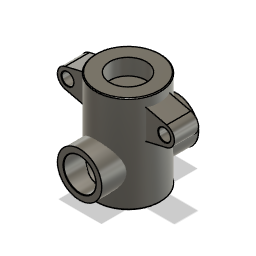
wheel hub v1 (Autodesk Fusion 360 design; units mm, degrees)
Autodesk Fusion 360 part; units mm, degrees
sketch "Sketch1" plane through (0, 0, 0) normal (0, 0, 1) x (1, 0, 0)
  line L0 (0, 0) -> (40, 0)
  line L1 (40, 0) -> (40, 120)
  line L2 (40, 120) -> (0, 120)
  line L3 (0, 120) -> (0, 0)
  dimension "d1" = 40
  dimension "d2" = 120
  constraint horizontal L0
  constraint vertical L1
  constraint horizontal L2
  constraint vertical L3
  constraint coincident L0.start L3.end
  measures "d1" distance of L1.end L2.end
  measures "d2" distance of L0.end L1.end
revolve "Revolve1" add sketch "Sketch1" angle 360 about axis through (0, 120, 0) along (0, -1, 0) makes body 1
sketch "Sketch2" plane through (0, 0, 0) normal (0, 0, 1) x (1, 0, 0)
sketch "Sketch3" plane through (0, 0, 0) normal (0, 0, 1) x (1, 0, 0)
  line L0 (0, 150) -> (0, -10) construction
  line L1 (-70, 90) -> (60, 90) construction
  line L2 (30, 110) -> (30, 70)
  line L3 (30, 70) -> (62.898, 77.8406)
  line L4 (30, 110) -> (62.898, 102.1594)
  circle A0 centre (60, 90) radius 7.5
  arc A1 (62.898, 77.8406) -> (62.898, 102.1594) centre (60, 90) ccw
  point P0 (40, 120)
  dimension "d4" = 25
  dimension "d5" = 20
  dimension "d6" = 40
  dimension "d7" = 10
  dimension "d8" = 15
  constraint vertical L0
  constraint perpendicular L0 L1
  constraint coincident L1.end A0.centre
  constraint perpendicular L1 L2
  constraint tangent L4 A1
  constraint tangent L3 A1
  constraint concentric A0 A1
  measures "d4" diameter of A1
  measures "d5" distance of L1 L2.start
  measures "d6" distance of L2.start L2.end
  measures "d7" horizontal distance of L2.start P0
  measures "d8" diameter of A0
extrude "Extrude1" add sketch "Sketch3" along normal blind 15 and the other way blind 15 separate body makes body 2
sketch "Sketch4" plane through (0, 0, 0) normal (0, 0, 1) x (1, 0, 0)
mirror "Mirror1" about plane through (0, 0, 0) normal (1, 0, 0) of bodies 2 makes body 3
sketch "Sketch5" plane through (0, 0, 0) normal (0, 0, 1) x (1, 0, 0)
  circle A0 centre (0, 40) radius 27.5
  line L0 (-40, 0) -> (40, 0)
  dimension "d15" = 55
  dimension "d16" = 40
  measures "d15" diameter of A0
  measures "d16" distance of A0.centre L0
extrude "Extrude2" add sketch "Sketch5" along normal blind 60 and the other way blind 60 separate body makes body 4
sketch "Sketch6" plane through (0, 0, 60) normal (0, 0, 1) x (1, 0, 0)
  circle A0 centre (0, 40) radius 27.5
  circle A1 centre (0, 40) radius 20
  dimension "d21" = 40
  constraint concentric A0 A1
  measures "d21" diameter of A1
extrude "Extrude3" cut sketch "Sketch6" along normal blind 60 and the other way blind 60 contours A1 bodies 1 4
sketch "Sketch7" plane through (0, 120, 0) normal (0, 1, 0) x (-1, 0, 0)
  circle A0 centre (0, 0) radius 40
  circle A1 centre (0, 0) radius 22.5
  dimension "d26" = 45
  constraint concentric A0 A1
  measures "d26" diameter of A1
extrude "Extrude4" cut 1 faces at (-6.8687, 44.386, 0) along direction (0, 0, 1) blind 60 and the other way blind 60 on bodies 4 bodies 1 4
extrude "Extrude5" cut sketch "Sketch7" along normal blind 0 and the other way blind 20 contours A1 bodies 1
fillet "Fillet1" radius 1 12 edges at (20, 40, 34.641) (20, 40, -34.641) (-37.2931, 0, -14.4646) (-37.2931, 120, -14.4646) (30, 90, 15) (30, 110, 0) (30, 90, -15) (30, 70, 0) (-30, 90, 15) (-30, 110, 0) (-30, 90, -15) (-30, 70, 0) 1 faces at (-23.3446, 53.6044, -32.4812) on bodies 1 2 3
chamfer "Chamfer1" distance 0.5 angle 45 6 edges at (53.0075, 92.7121, 15) (53.0075, 87.2879, -15) (-53.0075, 92.7121, 15) (-53.0075, 87.2879, -15) (-18.6465, 47.2323, 60) (-18.6465, 32.7677, -60) measured on face at (38.3212, 90, 15) measured on face at (38.3212, 90, -15) measured on face at (-67.4627, 89.2532, 5) measured on face at (-67.4627, 89.2532, 5) measured on face at (24.8232, 37.6402, 60) measured on face at (24.8232, 37.6402, -60) on bodies 2 3 4
